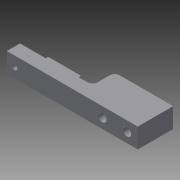
# Autodesk Inventor part: BottomWheelHolder
Saved by Autodesk Inventor 2015 (Build 190159000, 159)
## iProperties
Created: 2017-03-14
Part Number: BottomWheelHolder
Material: Generic
Document SubType Name: Modeling
Designer: 1esh9
Density: 1 g/cm^3
Appearance: Default
Author: 1esh9
Autodesk Inventor part; units mm, degrees
ref_plane "YZ Plane" through (0, 0, 0) normal (1, 0, 0) x (0, 1, 0)
ref_plane "XZ Plane" through (0, 0, 0) normal (0, 1, 0) x (-1, 0, 0)
ref_plane "XY Plane" through (0, 0, 0) normal (0, 0, 1) x (1, 0, 0)
sketch "Sketch1" plane through (0, 0, 0) normal (0, 0, 1) x (1, 0, 0)
  line L0 (0, 0) -> (79.43, 0)
  line L1 (79.43, 0) -> (79.43, -8)
  line L2 (79.43, -8) -> (0, -8)
  line L3 (0, -8) -> (0, 0)
  line L4 (79.43, 0) -> (43.93, 0)
  line L5 (43.93, 0) -> (43.93, 13.475)
  line L6 (43.93, 13.475) -> (79.43, 13.475)
  line L7 (79.43, 13.475) -> (79.43, 0)
  line L8 (3.2, 0) -> (6.4, 0) construction
  line L9 (6.4, 0) -> (6.4, -8) construction
  line L10 (6.4, -8) -> (3.2, -8) construction
  line L11 (3.2, -8) -> (3.2, 0) construction
  line L12 (4.8, 0) -> (4.8, -8) construction
  line L13 (55.93, 13.475) -> (55.93, -8) construction
  line L14 (70.93, 13.475) -> (70.93, -8) construction
  line L15 (53.43, 13.475) -> (58.43, 13.475) construction
  line L16 (58.43, 13.475) -> (58.43, -8) construction
  line L17 (58.43, -8) -> (53.43, -8) construction
  line L18 (53.43, -8) -> (53.43, 13.475) construction
  line L19 (68.43, 13.475) -> (73.43, 13.475) construction
  line L20 (73.43, 13.475) -> (73.43, -8) construction
  line L21 (73.43, -8) -> (68.43, -8) construction
  line L22 (68.43, -8) -> (68.43, 13.475) construction
  dimension "d0" = 13.475
  dimension "d3" = 3.2
  dimension "d4" = 3.2
  dimension "d6" = 39.13
  dimension "d34" = 8
  dimension "d35" = 5
  dimension "d36" = 5
  dimension "d37" = 2.5
  dimension "d38" = 2.5
  dimension "d39" = 12
  dimension "d40" = 10
  dimension "d41" = 6
  constraints: 46 end point, 10 parallel, 10 point on line, 7 perpendicular, 5 horizontal, 2 midpoint
  measures "d0" distance of L4.end L5.end
  measures "d3" distance between parallel lines of L9 L11
  measures "d4" distance between parallel lines of L3 L11
  measures "d6" distance between parallel lines of L5 L12
  measures "d34" distance of L2.end L0.start
  measures "d35" distance between parallel lines of L16 L18
  measures "d36" distance between parallel lines of L20 L22
  measures "d37" distance between parallel lines of L16 L13
  measures "d38" distance between parallel lines of L20 L14
  measures "d39" distance between parallel lines of L13 L5
  measures "d40" distance between parallel lines of L22 L16
  measures "d41" distance between parallel lines of L7 L20
extrude "Extrusion1" add sketch "Sketch1" along normal blind 12
sketch "Sketch2" plane through (43.93, 13.475, 0) normal (0, 1, 0) x (1, 0, 0)
  line L0 (35.5, 0) -> (0, 0) projected
  line L1 (0, 0) -> (0, -12) projected
  line L2 (35.5, -12) -> (0, -12) projected
  line L3 (35.5, 0) -> (35.5, -12) projected
  line L4 (0, 0) -> (0, -12) projected
  line L5 (0, 0) -> (-43.93, 0) projected
  line L6 (-43.93, 0) -> (-43.93, -12) projected
  line L7 (0, -12) -> (-43.93, -12) projected
  circle A0 centre (-39.13, -6) radius 1.6
  circle A1 centre (29, -6) radius 2.5
  circle A2 centre (14, -6) radius 2.5
  dimension "d15" = 3.2
  dimension "d16" = 5
  dimension "d17" = 5
  dimension "d22" = 12
  dimension "d23" = 6
  dimension "d24" = 6
  dimension "d26" = 3.2
  dimension "d42" = 14
  dimension "d43" = 10
  constraints: 3 centre point
  measures "d15" diameter of A0
  measures "d16" diameter of A2
  measures "d17" diameter of A1
  measures "d22" distance of L0.start L2.start
  measures "d23" distance from line of L2 A1.centre
  measures "d24" distance from line of L2 A2.centre
  measures "d26" distance edge to line of A0 L6
  measures "d42" distance from line of A2.centre L1
extrude "Extrusion2" cut sketch "Sketch2" against normal up to surface (21.475 mm away) contours A0 | A1 | A2
fillet "Fillet1" radius 3 2 edges at (43.93, 13.475, 6) (43.93, 0, 6)
sketch "Sketch3" plane through (0, 0, 12) normal (0, 1, 0) x (1, 0, 0)
  line L0 (40.93, 12) -> (40.93, 0) projected
  line L1 (40.93, 12) -> (0, 12) projected
  line L2 (0, 12) -> (0, 0) projected
  line L3 (40.93, 0) -> (0, 0) projected
  circle A0 centre (4.8, 6) radius 1.6 projected
  circle A1 centre (4.8, 6) radius 2.5
  circle A2 centre (4.8, 6) radius 1.6
  circle A3 centre (4.8, 6) radius 1.6 projected
  dimension "d31" = 5
  constraints: 2 centre point, 2 coincident, 1 concentric
  measures "d31" diameter of A1
extrude "Extrusion3" add sketch "Sketch3" along normal blind 0.5 contours A1
sketch "Sketch4" plane through (0, 0, 12) normal (0, 1, 0) x (1, 0, 0)
  line L0 (43.93, 0) -> (43.93, 12) projected
  line L1 (43.93, 12) -> (43.93, 0) projected
  circle A0 centre (4.8, 6) radius 2.5 projected
  line L2 (40.93, 12) -> (40.93, 0) projected
  line L3 (40.93, 12) -> (0, 12) projected
  line L4 (0, 12) -> (0, 0) projected
  line L5 (40.93, 0) -> (0, 0) projected
  line L6 (43.93, 12) -> (43.93, 0) projected
  line L7 (43.93, 0) -> (43.93, 12) projected
  line L8 (0, 12) -> (79.43, 12) projected
  line L9 (15.63, 12) -> (35.63, 12)
  line L10 (35.63, 12) -> (35.63, 0)
  line L11 (35.63, 0) -> (15.63, 0)
  line L12 (15.63, 0) -> (15.63, 12)
  dimension "d44" = 8.3
  dimension "d45" = 20
  constraints: 8 end point, 2 parallel, 2 point on line, 1 horizontal, 1 perpendicular
  measures "d44" distance from line of L0.start L10
  measures "d45" distance between parallel lines of L10 L12
extrude "Extrusion4" add sketch "Sketch4" along normal blind 1.5 contours L10 L5 L12 L3
equation "\"d37\" = 0.5 * d35"
equation "\"d38\" = 0.5 * d36"
body "Solid1"
